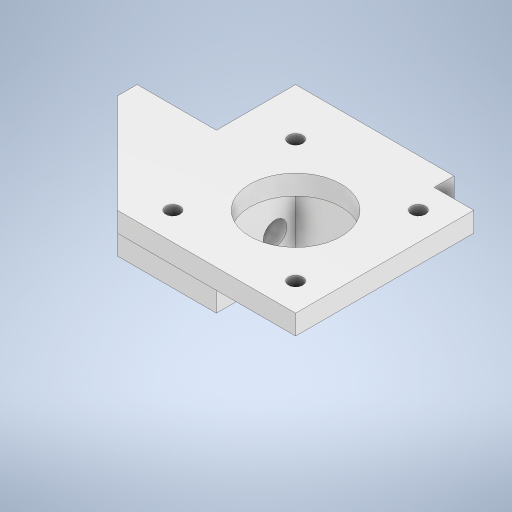
# Autodesk Inventor part: NEMA17 Stepper CornerMount
Saved by Autodesk Inventor 2023 (Build 270158000, 158)
## iProperties
Created: 2023-04-11
Part Number: NEMA17 Stepper CornerMount
Material: PC/ABS Plastic
Document SubType Name: Modeling
Designer: ethan
Density: 0.357273 g/cm^3
Appearance: Smooth - White
Author: ethan
Autodesk Inventor part; units mm, degrees
ref_plane "YZ Plane" through (0, 0, 0) normal (1, 0, 0) x (0, 1, 0)
ref_plane "XZ Plane" through (0, 0, 0) normal (0, 1, 0) x (-1, 0, 0)
ref_plane "XY Plane" through (0, 0, 0) normal (0, 0, 1) x (1, 0, 0)
sketch "Sketch1" plane through (0, 0, 0) normal (0, 1, 0) x (-1, 0, 0)
  line L0 (0, 0) -> (-31, 0) construction
  line L1 (-31, 0) -> (-31, -31) construction
  line L2 (-31, -31) -> (0, -31) construction
  line L3 (0, -31) -> (0, 0) construction
  circle A0 centre (0, 0) radius 1.8
  circle A1 centre (0, -31) radius 1.8
  circle A2 centre (-31, -31) radius 1.8
  circle A3 centre (-31, 0) radius 1.8
  line L4 (-38, 7) -> (-38, -38)
  line L5 (-38, -38) -> (7, -38)
  line L6 (7, 7) -> (-38, -38) construction
  line L7 (-38, 7) -> (7, -38) construction
  circle A4 centre (-15.5, -15.5) radius 11.5
  line L8 (7, 7) -> (-38, 7)
  line L9 (7, -38) -> (7, 7)
  line L10 (7, -43) -> (12, -43)
  line L11 (12, -43) -> (12, -18)
  line L12 (12, -18) -> (7, -18)
  line L13 (7, -18) -> (7, -43)
  line L14 (12, -18) -> (32, -18)
  line L15 (32, -18) -> (32, -23)
  line L16 (32, -23) -> (12, -23)
  line L17 (12, -23) -> (12, -18)
  line L18 (7, -38) -> (-28, -38)
  line L19 (-28, -38) -> (-28, -43)
  line L20 (-28, -43) -> (7, -43)
  line L21 (7, -43) -> (7, -38)
  point P0 (7, -38)
  point P1 (7, -38)
  dimension "d0" = 31
  dimension "d1" = 31
  dimension "d2" = 3.6
  dimension "d3" = 3.6
  dimension "d4" = 3.6
  dimension "d5" = 3.6
  dimension "d17" = 23
  dimension "d18" = 45
  dimension "d19" = 45
  dimension "d37" = 5
  dimension "d38" = 25
  dimension "d39" = 20
  dimension "d40" = 5
  dimension "d42" = 5
  dimension "d43" = 35
  constraints: 44 end point, 8 parallel, 6 perpendicular, 5 centre point, 5 horizontal, 4 coincident, 3 point on line, 1 midpoint
  measures "d0" distance of L2.end L1.end
  measures "d1" distance of L1.end L0.end
  measures "d2" diameter of A0
  measures "d3" diameter of A3
  measures "d4" diameter of A2
  measures "d5" diameter of A1
  measures "d17" diameter of A4
  measures "d18" distance between parallel lines of L8 L5
  measures "d19" distance from line of L4 L5.end
  measures "d37" distance of L12.end L11.end
  measures "d38" distance of L11.end L10.end
  measures "d39" distance of L15.end L16.end
  measures "d40" distance of L14.end L15.end
  measures "d42" distance between parallel lines of L5 L10
  measures "d43" distance of L10.start L19.end
extrude "Extrusion1" add sketch "Sketch1" against normal blind 5 contours L8 L9 L5 L4
extrude "Extrusion4" add sketch "Sketch1" against normal blind 35 contours L5 L13 L20 L19 | L12 L11 L10 L13 L9 | L14 L15 L16 L11
chamfer "Chamfer1" distance 30 angle 45 1 edges at (28, -35, -40.5)
chamfer "Chamfer2" distance 25 angle 45 1 edges at (-7, -2.5, -18)
sketch "Sketch3" plane through (-12, 0, -43) normal (-1, 0, 0) x (0, 0, 1)
  line L0 (10.2, 0) -> (13.8, 0) construction
  line L1 (10.2, 0) -> (10.2, -35) construction
  line L2 (5, -35) -> (25, -35) construction
  circle A0 centre (10.2, -25) radius 3
  line L3 (20, -35) -> (0, -35) projected
  line L4 (0, 0) -> (20, 0) projected
  point P0 (43, 0)
  dimension "d51" = 6
  dimension "d55" = 10
  constraints: 2 end point, 2 point on line, 1 centre point, 1 vertical
  measures "d51" diameter of A0
  measures "d55" distance from line of L3 A0.centre
extrude "Extrusion5" cut sketch "Sketch3" against normal blind 5
sketch "Sketch4" plane through (-12, 0, -23) normal (0, 0, -1) x (-1, 0, 0)
  line L0 (0, 0) -> (20, 0) construction
  line L1 (10, 0) -> (10, -35) construction
  line L2 (20, -35) -> (0, -35) construction
  circle A0 centre (10, -10) radius 3
  circle A1 centre (10, -25) radius 3
  point P0 (-12, 0)
  dimension "d58" = 6
  dimension "d59" = 6
  dimension "d60" = 10
  dimension "d61" = 10
  constraints: 2 centre point, 2 end point, 2 midpoint, 2 point on line
  measures "d58" diameter of A0
  measures "d59" diameter of A1
  measures "d60" distance from line of L0 A0.centre
  measures "d61" distance from line of L2 A1.centre
extrude "Extrusion6" cut sketch "Sketch4" against normal blind 5
equation "\"d3\" = d2"
equation "\"d4\" = d2"
equation "\"d5\" = d2"
body "Solid1"
